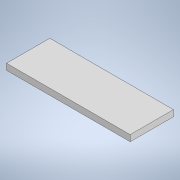
# Autodesk Inventor part: Cover
Saved by Autodesk Inventor 2021 (Build 250183000, 183)
## iProperties
Created: 2020-06-27
Part Number: Cover
Material: Generic
Document SubType Name: Modeling
Designer: Mariano
Density: 1 g/cm^3
Appearance: Default
Author: Mariano
Autodesk Inventor part; units mm, degrees
ref_plane "YZ Plane" through (0, 0, 0) normal (1, 0, 0) x (0, 1, 0)
ref_plane "XZ Plane" through (0, 0, 0) normal (0, 1, 0) x (-1, 0, 0)
ref_plane "XY Plane" through (0, 0, 0) normal (0, 0, 1) x (1, 0, 0)
sketch "Sketch1" plane through (0, 0, 0) normal (0, 1, 0) x (-1, 0, 0)
  line L0 (20, 7) -> (-20, 7)
  line L1 (-20, 7) -> (-20, -7)
  line L2 (-20, -7) -> (20, -7)
  line L3 (20, -7) -> (20, 7)
  line L4 (20, 7) -> (-20, -7) construction
  line L5 (-20, 7) -> (20, -7) construction
  point P0 (0, 0)
  dimension "d0" = 14
  dimension "d1" = 40
  constraints: 12 end point, 2 midpoint, 2 parallel, 1 horizontal, 1 perpendicular
  measures "d0" distance of L0.end L1.end
  measures "d1" distance of L1.end L2.end
extrude "Extrusion1" add sketch "Sketch1" along normal blind 2
body "Solid1"
